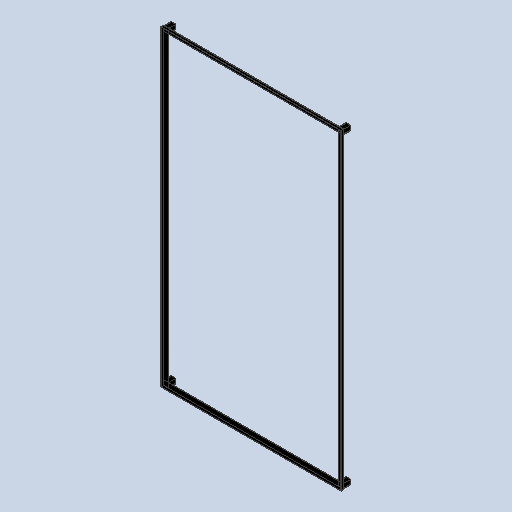
# Autodesk Inventor part: estruturaMesa
Saved by Autodesk Inventor 2025 (Build 290162000, 162)
## iProperties
Created: 2022-08-16
Part Number: estruturaMesa
Material: Generic
Document SubType Name: Modeling
Designer: cvss2
Density: 1 g/cm^3
Appearance: Default
Author: cvss2
Autodesk Inventor part; units mm, degrees
ref_plane "YZ Plane" through (0, 0, 0) normal (1, 0, 0) x (0, 1, 0)
ref_plane "XZ Plane" through (0, 0, 0) normal (0, 1, 0) x (-1, 0, 0)
ref_plane "XY Plane" through (0, 0, 0) normal (0, 0, 1) x (1, 0, 0)
sketch "Sketch1" plane through (0, 0, 0) normal (0, 0, 1) x (1, 0, 0)
  line L0 (0, 0) -> (-1500, 0)
  line L1 (-1500, 0) -> (-1500, -2600)
  line L2 (-1500, -2600) -> (0, -2600)
  line L3 (0, -2600) -> (0, 0)
  line L4 (-40, -40) -> (-1460, -40)
  line L5 (-1460, -40) -> (-1460, -2560)
  line L6 (-1460, -2560) -> (-40, -2560)
  line L7 (-40, -2560) -> (-40, -40)
  dimension "d0" = 1500
  dimension "d1" = 2600
  dimension "d2" = 40
  constraints: 16 end point, 4 parallel, 2 perpendicular, 1 horizontal, 3 other
  measures "d0" distance of L2.end L1.end
  measures "d1" distance of L1.end L0.end
  measures "d2" distance between parallel lines of L3 L7
extrude "Extrusion1" add sketch "Sketch1" along normal blind 20
shell "Shell1" thickness 3 outward yes removed faces 5 at (-1486.6667, -880, 20) at (-1460, -1720, 6.6667) at (-40, -880, 6.6667) at (-513.3333, -2560, 13.3333) at (-986.6667, -40, 13.3333)
sketch "Sketch2" plane through (0, 0, -3) normal (0, 0, -1) x (-1, 0, 0)
  line L0 (1503, 3) -> (1503, -2603) projected
  line L1 (-3, 3) -> (1503, 3) projected
  line L2 (-3, -2603) -> (-3, 3) projected
  line L3 (1503, -2603) -> (-3, -2603) projected
  line L4 (40, -40) -> (40, -2560) projected
  line L5 (1460, -40) -> (40, -40) projected
  line L6 (1460, -2560) -> (1460, -40) projected
  line L7 (40, -2560) -> (1460, -2560) projected
  line L8 (1460, -2560) -> (1460, -40) projected
  line L9 (1500, -2600) -> (0, -2600) projected
  line L10 (1460, -2560) -> (1500, -2560)
  line L11 (1500, -2560) -> (1500, -2600)
  line L12 (1500, -2600) -> (1460, -2600)
  line L13 (1460, -2600) -> (1460, -2560)
  line L14 (0, -2600) -> (0, -2560)
  line L15 (40, -2560) -> (40, -2600)
  line L16 (40, -2600) -> (0, -2600)
  line L17 (0, -2560) -> (40, -2560)
  line L18 (1460, -40) -> (1460, 0)
  line L19 (1500, 0) -> (1500, -40)
  line L20 (1500, -40) -> (1460, -40)
  line L21 (1460, 0) -> (1500, 0)
  line L22 (0, -40) -> (0, 0)
  line L23 (40, 0) -> (40, -40)
  line L24 (40, -40) -> (0, -40)
  line L25 (0, 0) -> (40, 0)
  point P0 (0, 0)
  dimension "d8" = 1460
  dimension "d11" = 2560
  constraints: 32 end point, 2 horizontal, 2 parallel, 1 perpendicular, 1 vertical, 24 other
  measures "d8" distance of L12.end L14.start
  measures "d11" distance of L12.end L18.start
extrude "Extrusion2" add sketch "Sketch2" along normal blind 60 separate body contours L18 L21 L19 L20 | L24 L22 L25 L23 | L15 L9 L14 L17 | L10 L11 L9 L13
shell "Shell2" thickness 3 removed faces 4 at (-1486.6667, -13.3333, -63) at (-1486.6667, -2573.3333, -63) at (-26.6667, -2573.3333, -63) at (-13.3333, -13.3333, -63) bodies 2
equation "\"d0\" = comprimento"
equation "\"d1\" = largura"
equation "\"comprimento\" = 1500"
equation "\"largura\" = 2600"
body "Solid1"
body "Solid2"
